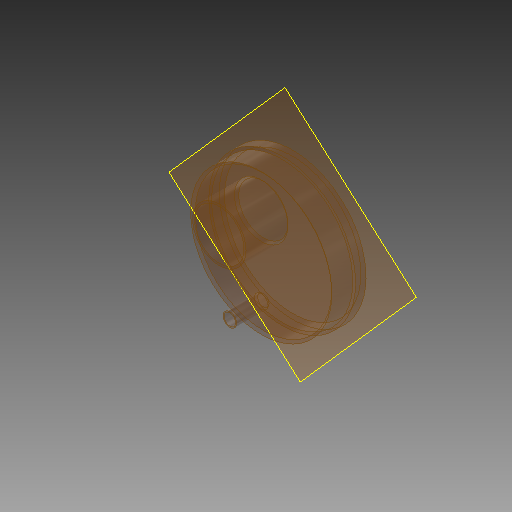
# Autodesk Inventor part: Tampa de Entrada
Saved by Autodesk Inventor 2019 (Build 230136000, 136)
## iProperties
Created: 2020-04-02
Part Number: Tampa de Entrada
Material: Genérico
Document SubType Name: Modeling
Designer: Paulo Rodrigues
Density: 1 g/cm^3
Appearance: Policarbonato - Fumê
Author: Paulo Rodrigues
Autodesk Inventor part; units mm, degrees
ref_plane "YZ Plane" through (0, 0, 0) normal (1, 0, 0) x (0, 1, 0)
ref_plane "XZ Plane" through (0, 0, 0) normal (0, 1, 0) x (-1, 0, 0)
ref_plane "XY Plane" through (0, 0, 0) normal (0, 0, 1) x (1, 0, 0)
ref_plane "Plano de trabalho1" through (12.8418, -28.4792, 0) normal (0, 0, 1) x (0.6621, 0.7495, 0)
sketch "Esboço1" plane through (12.8418, -28.4792, 0) normal (0, 0, 1) x (0.6621, 0.7495, 0)
  circle A0 centre (38, 0) radius 32.5 projected
  circle A1 centre (38, 0) radius 35
  point P0 (12.8418, 28.4792)
  dimension "d0" = 70
  constraints: 1 centre point, 1 coincident
  measures "d0" diameter of A1
extrude "Extrusão1" add sketch "Esboço1" along normal blind 5
sketch "Esboço2" plane through (38, 0, 5) normal (0, 0, 1) x (1, 0, 0)
  circle A0 centre (0, 0) radius 34.6774 projected
  circle A1 centre (0, 0) radius 32.5 projected
  circle A2 centre (0, 0) radius 33.6774
  point P0 (-38, 0)
  dimension "d3" = 1
  constraints: 1 centre point
  measures "d3" radial gap between concentric circles of A0 A2
extrude "Extrusão2" add sketch "Esboço2" along normal blind 10 contours A2
sketch "Esboço3" plane through (38, 0, 15) normal (0, 0, 1) x (1, 0, 0)
  circle A0 centre (0, 0) radius 32.5 projected
  point P0 (-38, 0)
extrude "Extrusão3" add sketch "Esboço3" against normal blind 1
sketch "Esboço4" plane through (38, 0, 15) normal (0, 0, 1) x (1, 0, 0)
  circle A0 centre (0, 0) radius 33.6774 projected
  circle A1 centre (0, 17.5016) radius 12.75
  circle A2 centre (0, 17.5016) radius 11.75
  point P0 (-38, 0)
  dimension "d8" = 25.5
  dimension "d9" = 1
  constraints: 2 centre point
  measures "d8" diameter of A1
  measures "d9" radial gap between concentric circles of A1 A2
extrude "Extrusão4" add sketch "Esboço4" along normal blind 20 contours A1
sketch "Esboço5" plane through (38, 0, 15) normal (0, 0, 1) x (1, 0, 0)
  circle A0 centre (0, 0) radius 33.6774 projected
  circle A1 centre (0, 17.5016) radius 12.75 projected
  circle A2 centre (0, -20) radius 3.25
  circle A3 centre (0, -20) radius 2.75
  point P0 (-38, 0)
  dimension "d12" = 6.5
  dimension "d14" = 0.5
  dimension "d15" = 20
  constraints: 2 centre point
  measures "d12" diameter of A2
  measures "d14" radial gap between concentric circles of A2 A3
  measures "d15" distance of A0.centre A2.centre
extrude "Extrusão5" add sketch "Esboço5" along normal blind 15 contours A2
sketch "Esboço6" plane through (38, 0, 15) normal (0, 0, 1) x (1, 0, 0)
  circle A0 centre (0, -20) radius 2.75 projected
  circle A1 centre (0, 17.5016) radius 11.75 projected
  point P0 (-38, 0)
extrude "Extrusão6" cut sketch "Esboço6" against normal blind 15
